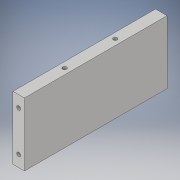
# Autodesk Inventor part: BatterySide
Saved by Autodesk Inventor 2019 (Build 230136000, 136)
## iProperties
Created: 2018-11-18
Part Number: BatterySide
Material: Generic
Document SubType Name: Modeling
Designer: james
Density: 1 g/cm^3
Appearance: Default
Author: james
Autodesk Inventor part; units mm, degrees
ref_plane "YZ Plane" through (0, 0, 0) normal (1, 0, 0) x (0, 1, 0)
ref_plane "XZ Plane" through (0, 0, 0) normal (0, 1, 0) x (-1, 0, 0)
ref_plane "XY Plane" through (0, 0, 0) normal (0, 0, 1) x (1, 0, 0)
sketch "Sketch1" plane through (0, 0, 0) normal (0, 1, 0) x (-1, 0, 0)
  line L0 (7.0328, 27.6191) -> (-5.6672, 27.6191)
  line L1 (-5.6672, 27.6191) -> (-5.6672, -129.8609)
  line L2 (-5.6672, -129.8609) -> (7.0328, -129.8609)
  line L3 (7.0328, -129.8609) -> (7.0328, 27.6191)
  point P0 (0, 0)
  dimension "d0" = 12.7
  dimension "d1" = 157.48
  constraints: 8 end point, 2 parallel, 1 horizontal, 1 perpendicular
  measures "d0" distance of L0.start L0.end
  measures "d1" distance of L2.end L0.start
extrude "Extrusion1" add sketch "Sketch1" along normal blind 69.85
sketch "Sketch2" plane through (-7.0328, 0, 27.6191) normal (0, 0, 1) x (1, 0, 0)
  line L0 (12.7, 0) -> (12.7, 69.85) projected
  line L1 (12.7, 0) -> (0, 0) projected
  line L2 (0, 69.85) -> (12.7, 69.85) projected
  point P0 (7.0328, 0)
  point P1 (6.35, 57.15)
  point P2 (6.35, 12.7)
  dimension "d4" = 0
  dimension "d5" = 6.35
  dimension "d6" = 12.7
  dimension "d7" = 12.7
  measures "d4" horizontal distance of point (6.35, 12.7) point (6.35, 57.15)
  measures "d5" distance from line of L0 point (6.35, 12.7)
  measures "d6" distance from line of L1 point (6.35, 12.7)
  measures "d7" distance from line of L2 point (6.35, 57.15)
hole "Hole1" at (-0.6828, 57.15, 27.6191) at (-0.6828, 12.7, 27.6191) direction (0, 0, -1) diameter 4.318 end through all
sketch "Sketch3" plane through (0, 69.85, 0) normal (0, 1, 0) x (1, 0, 0)
  line L0 (-7.0328, 129.8609) -> (-7.0328, -27.6191) projected
  line L1 (-7.0328, -27.6191) -> (5.6672, -27.6191) projected
  line L2 (5.6672, 129.8609) -> (-7.0328, 129.8609) projected
  point P0 (0, 0)
  point P1 (-0.6828, 23.1809)
  point P2 (-0.6828, 23.0627)
  point P3 (-0.6828, 79.0609)
  dimension "d15" = 0
  dimension "d16" = 6.35
  dimension "d17" = 50.8
  dimension "d18" = 50.8
  dimension "d26" = 55.88
  measures "d15" horizontal distance of point (-0.683, 23.181) point (-0.683, 23.063)
  measures "d16" distance from line of L0 point (-0.683, 23.181)
  measures "d17" distance from line of L1 point (-0.683, 23.181)
  measures "d18" distance from line of L2 point (-0.683, 79.061)
  measures "d26" distance of point (-0.683, 23.181) point (-0.683, 79.061)
hole "Hole2" at (-0.6828, 69.85, -23.1809) at (-0.6828, 69.85, -23.0627) at (-0.6828, 69.85, -79.0609) direction (0, -1, 0) diameter 4.318 end through all
body "Solid1"
